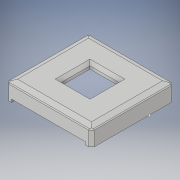
# Autodesk Inventor part: Raspberrycamhalter oberteil
Saved by Autodesk Inventor 2017 (Build 210142000, 142)
## iProperties
Part Number: Raspberrycamhalter oberteil
Material: Generisch
Document SubType Name: Modeling
Designer: pgmadmin
Density: 1 g/cm^3
Appearance: Vorgabe
Author: pgmadmin
Autodesk Inventor part; units mm, degrees
ref_plane "YZ Plane" through (0, 0, 0) normal (1, 0, 0) x (0, 1, 0)
ref_plane "XZ Plane" through (0, 0, 0) normal (0, 1, 0) x (-1, 0, 0)
ref_plane "XY Plane" through (0, 0, 0) normal (0, 0, 1) x (1, 0, 0)
sketch "Skizze1" plane through (0, 0, 0) normal (0, 0, 1) x (1, 0, 0)
  line L0 (-7.9625, 6.5659) -> (17.5375, 6.5659)
  line L1 (17.5375, 6.5659) -> (17.5375, -17.9341)
  line L2 (17.5375, -17.9341) -> (-7.9625, -17.9341)
  line L3 (-7.9625, -17.9341) -> (-7.9625, 6.5659)
  line L4 (-9.9625, 8.5659) -> (19.5375, 8.5659)
  line L5 (19.5375, 8.5659) -> (19.5375, -19.9341)
  line L6 (19.5375, -19.9341) -> (-9.9625, -19.9341)
  line L7 (-9.9625, -19.9341) -> (-9.9625, 8.5659)
  point P0 (0, 0)
  dimension "d0" = 25.5
  dimension "d1" = 24.5
  dimension "d2" = 2
  dimension "d3" = 2
  dimension "d4" = 2
  dimension "d5" = 2
  constraints: 16 end point, 4 parallel, 2 horizontal, 2 perpendicular
  measures "d0" distance of L1.end L2.end
  measures "d1" distance of L0.end L1.end
  measures "d2" distance between parallel lines of L3 L7
  measures "d3" distance between parallel lines of L0 L4
  measures "d4" distance between parallel lines of L5 L1
  measures "d5" distance between parallel lines of L6 L2
extrude "Extrusion1" add sketch "Skizze1" along normal blind 4
sketch "Skizze2" plane through (0, 0, 4) normal (0, 0, 1) x (1, 0, 0)
  line L0 (-9.9625, -19.9341) -> (19.5375, -19.9341) projected
  line L1 (-9.9625, 8.5659) -> (19.5375, 8.5659)
  line L2 (19.5375, 8.5659) -> (19.5375, -19.9341)
  line L3 (19.5375, -19.9341) -> (-9.9625, -19.9341)
  line L4 (-9.9625, -19.9341) -> (-9.9625, 8.5659)
  point P0 (0, 0)
  constraints: 8 end point, 2 parallel, 1 horizontal, 1 perpendicular
extrude "Extrusion2" add sketch "Skizze2" along normal blind 2
chamfer "Fase1" distance 1 angle 45 8 edges at (4.7875, 8.5659, 6) (-9.9625, -5.6841, 6) (-9.9625, 8.5659, 3) (19.5375, 8.5659, 3) (19.5375, -5.6841, 6) (4.7875, -19.9341, 6) (19.5375, -19.9341, 3) (-9.9625, -19.9341, 3)
chamfer "Fase2" distance 1 angle 45 4 edges at (18.5375, -5.6841, 6) (4.7875, 7.5659, 6) (-8.9625, -5.6841, 6) (4.7875, -18.9341, 6)
sketch "Skizze3" plane through (0, 0, 4) normal (0, 0, -1) x (-1, 0, 0)
  line L0 (-9.5375, -0.4341) -> (0.4625, -0.4341)
  line L1 (0.4625, -0.4341) -> (0.4625, -10.4341)
  line L2 (0.4625, -10.4341) -> (-9.5375, -10.4341)
  line L3 (-9.5375, -10.4341) -> (-9.5375, -0.4341)
  line L4 (-17.5375, 6.5659) -> (7.9625, 6.5659) projected
  line L5 (7.9625, -17.9341) -> (7.9625, 6.5659) projected
  line L6 (-17.5375, 6.5659) -> (-17.5375, -17.9341) projected
  line L7 (-17.5375, -17.9341) -> (7.9625, -17.9341) projected
  point P0 (0, 0)
  dimension "d16" = 10
  dimension "d17" = 10
  dimension "d18" = 7
  dimension "d19" = 7.5
  dimension "d20" = 8
  dimension "d21" = 7.5
  constraints: 8 end point, 2 parallel, 1 horizontal, 1 perpendicular
  measures "d16" distance between parallel lines of L3 L1
  measures "d17" distance between parallel lines of L0 L2
  measures "d18" distance between parallel lines of L4 L0
  measures "d19" distance between parallel lines of L5 L1
  measures "d20" distance between parallel lines of L6 L3
  measures "d21" distance between parallel lines of L7 L2
extrude "Extrusion3" cut sketch "Skizze3" against normal blind 67 contours L0 L1 L2 L3
chamfer "Fase3" distance 1 angle 45 4 edges at (4.5375, -0.4341, 6) (-0.4625, -5.4341, 6) (9.5375, -5.4341, 6) (4.5375, -10.4341, 6)
sketch "Skizze4" plane through (0, 0, 0) normal (0, 0, -1) x (-1, 0, 0)
  line L0 (-17.5375, -17.9341) -> (7.9625, -17.9341) projected
  line L1 (-17.5375, -17.9341) -> (8.0395, -17.9341)
  line L2 (8.0395, -17.9341) -> (8.0395, -21.0501)
  line L3 (8.0395, -21.0501) -> (-17.5375, -21.0501)
  line L4 (-17.5375, -21.0501) -> (-17.5375, -17.9341)
  point P0 (0, 0)
  constraints: 8 end point, 2 parallel, 1 horizontal, 1 perpendicular
extrude "Extrusion4" cut sketch "Skizze4" against normal blind 1
sketch "Skizze5" plane through (19.5375, -18.9341, 0) normal (1, 0, 0) x (0, 0, -1)
  point P0 (0, 18.9341)
